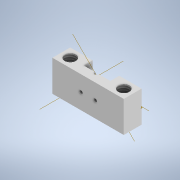
# Autodesk Inventor part: air delivery
Saved by Autodesk Inventor 2021.2 (Build 252289000, 289)
## iProperties
Created: 2021-07-12
Part Number: air delivery
Material: Generic
Document SubType Name: Modeling
Designer: jl4459
Density: 1 g/cm^3
Appearance: Default
Author: jl4459
Autodesk Inventor part; units mm, degrees
ref_plane "YZ Plane" through (0, 0, 0) normal (1, 0, 0) x (0, 1, 0)
ref_plane "XZ Plane" through (0, 0, 0) normal (0, 1, 0) x (-1, 0, 0)
ref_plane "XY Plane" through (0, 0, 0) normal (0, 0, 1) x (1, 0, 0)
sketch "Sketch1" plane through (0, 0, 0) normal (0, 1, 0) x (-1, 0, 0)
  line L0 (12.7, 3.175) -> (-12.7, 3.175)
  line L1 (-12.7, 3.175) -> (-12.7, -3.175)
  line L2 (12.7, -3.175) -> (12.7, 3.175)
  line L3 (4.7625, 0) -> (-4.7625, 0)
  line L4 (-4.7625, 0) -> (-4.7625, -3.175)
  line L5 (4.7625, 0) -> (4.7625, -3.175)
  line L6 (12.7, -3.175) -> (4.7625, -3.175)
  line L7 (-4.7625, -3.175) -> (-12.7, -3.175)
  point P0 (0, 0)
  dimension "d0" = 25.4
  dimension "d1" = 6.35
  dimension "d2" = 9.525
  constraints: 16 end point, 2 equal length, 2 horizontal, 2 perpendicular
  measures "d0" distance of L2.start L1.end
  measures "d1" distance of L1.end L0.end
  measures "d2" distance of L3.start L3.end
extrude "Extrusion1" add sketch "Sketch1" along normal blind 11.1125
sketch "Sketch2" plane through (0, 11.1125, 0) normal (0, 1, 0) x (1, 0, 0)
  line L0 (12.7, -3.175) -> (12.7, 3.175) projected
  line L1 (-12.7, 3.175) -> (-12.7, -3.175) projected
  point P0 (0, 0)
  point P1 (9.525, 0)
  point P2 (-9.525, 0)
  dimension "d5" = 3.175
  dimension "d6" = 3.175
  measures "d5" distance from line of point (9.525, 0) L0
  measures "d6" distance from line of L1 point (-9.525, 0)
hole "Hole1" at (-10.16, 0, 0) direction (0.7071068, 0.7071068, 0) diameter 1.27 depth 2.54 start extended yes
hole "Hole3" at (10.16, 0, 0) direction (-0.7071068, 0.7071068, 0) diameter 1.27 depth 2.54 start extended yes
hole "Hole2" at (-9.525, 11.1125, 0) at (9.525, 11.1125, 0) direction (0, -1, 0) diameter 3.9624 depth 6.35 start extended yes thread size "10-32 UNF" class "2B" standard "ANSI Unified Screw Threads"
sketch "Sketch6" plane through (9.525, 4.7625, 0) normal (0, 1, 0) x (1, 0, 0)
  line L0 (3.175, -3.175) -> (3.175, 3.175) projected
  point P0 (-9.525, 0)
  point P1 (-0.635, 0.0383)
  dimension "d42" = 3.81
  measures "d42" distance from line of L0 point (-0.635, 0.038)
hole "Hole4" at (8.89, 4.7625, -0.0383) direction (0, -1, 0) diameter 1.27 depth 3.683 start extended yes
sketch "Sketch7" plane through (-9.525, 4.7625, 0) normal (0, 1, 0) x (1, 0, 0)
  line L0 (-3.175, 3.175) -> (-3.175, -3.175) projected
  point P0 (9.525, 0)
  point P1 (0.635, 0.0249)
  dimension "d52" = 3.81
  measures "d52" distance from line of L0 point (0.635, 0.025)
hole "Hole5" at (-8.89, 4.7625, -0.0249) direction (0, -1, 0) diameter 1.27 depth 3.683 start extended yes
sketch "Sketch8" plane through (4.7625, 0, 0) normal (0, 0, -1) x (-1, 0, 0)
  line L0 (17.4625, 0) -> (17.4625, 11.1125) projected
  line L1 (-7.9375, 0) -> (-7.9375, 11.1125) projected
  point P0 (4.7625, 0)
  point P1 (2.2225, 5.5563)
  point P2 (7.3025, 5.5563)
  dimension "d64" = 10.16
  dimension "d65" = 10.16
  measures "d64" distance from line of L0 point (7.303, 5.556)
  measures "d65" distance from line of L1 point (2.223, 5.556)
hole "Hole6" at (-2.54, 5.5563, 0) at (2.54, 5.5563, 0) direction (0, 0, 1) diameter 1.1811 depth 4.6482 start extended yes thread size "0-80 UNF" class "2B" standard "ANSI Unified Screw Threads"
sketch "Sketch9" plane through (0, 0, 0) normal (0, -1, 0) x (1, 0, 0)
  line L0 (12.7, 3.175) -> (12.7, -3.175) projected
  line L1 (4.7625, 0) -> (-4.7625, 0) projected
  point P0 (0, 0)
  point P1 (0, 0.1905)
  dimension "d73" = 12.7
  dimension "d81" = 0.1905
  measures "d73" distance from line of L0 point (0, 0.191)
  measures "d81" distance from line of L1 point (0, 0.191)
hole "Hole7" at (0, 0, 0.1905) direction (0, 1, 0) diameter 1.27 end through all start extended yes
body "Solid1"
